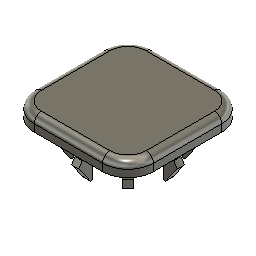
hole plug (Autodesk Fusion 360 design; units mm, degrees)
Autodesk Fusion 360 part; units mm, degrees
note: some values were not read from the file. Set by a fixed rule: which face or edge a step refers to.
sketch "Sketch1" plane through (0, 0, 0) normal (0, 1, 0) x (1, 0, 0)
  line L0 (0, 0) -> (16.4, 0)
  line L1 (16.4, 0) -> (16.4, -16.4)
  line L2 (16.4, -16.4) -> (0, -16.4)
  line L3 (0, -16.4) -> (0, 0)
  line L4 (0, 0) -> (55.9566, 0)
  line L5 (0, 0) -> (0, 56.0794)
  line L6 (-16.4, -16.4) -> (0, -16.4)
  line L7 (-16.4, 0) -> (-16.4, -16.4)
  line L8 (16.4, 0) -> (16.4, 16.4)
  line L9 (16.4, 16.4) -> (0, 16.4)
  line L10 (-16.4, 16.4) -> (0, 16.4)
  line L11 (-16.4, 0) -> (-16.4, 16.4)
  circle A0 centre (0, 0) radius 13.6
  circle A1 centre (0, 0) radius 14.6
  circle A2 centre (0, 0) radius 10.75
  line L12 (0, 0) -> (-10.3238, -10.3238) construction
  line L13 (0, 0) -> (0, -14.6) construction
  line L14 (0, 0) -> (10.3238, -10.3238) construction
  line L15 (0, 0) -> (14.6, 0) construction
  line L16 (0, 0) -> (10.3238, 10.3238) construction
  line L17 (0, 0) -> (0, 14.6) construction
  line L18 (0, 0) -> (-10.3238, 10.3238) construction
  line L19 (0, 0) -> (-14.6, 0) construction
  line L20 (-11.0066, -9.5924) -> (-8.2755, -6.8613)
  line L21 (-9.5924, -11.0066) -> (-6.8613, -8.2755)
  line L22 (1, -14.5657) -> (1, -10.7034)
  line L23 (-1, -14.5657) -> (-1, -10.7034)
  line L24 (11.0066, -9.5924) -> (8.2755, -6.8613)
  line L25 (9.5924, -11.0066) -> (6.8613, -8.2755)
  line L26 (14.5657, 1) -> (10.7034, 1)
  line L27 (14.5657, -1) -> (10.7034, -1)
  line L28 (9.5924, 11.0066) -> (6.8613, 8.2755)
  line L29 (11.0066, 9.5924) -> (8.2755, 6.8613)
  line L30 (-1, 14.5657) -> (-1, 10.7034)
  line L31 (1, 14.5657) -> (1, 10.7034)
  line L32 (-11.0066, 9.5924) -> (-8.2755, 6.8613)
  line L33 (-9.5924, 11.0066) -> (-6.8613, 8.2755)
  line L34 (-14.5657, -1) -> (-10.7034, -1)
  line L35 (-14.5657, 1) -> (-10.7034, 1)
  dimension "d3" = 32.8
  dimension "d5" = 32.8
  dimension "d6" = 27.2
  dimension "d7" = 29.2
  dimension "d8" = 21.5
  dimension "d10" = 360
  dimension "d11" = 1
  dimension "d12" = 1
  dimension "d14" = 360
  constraint horizontal L0
  constraint vertical L1
  constraint horizontal L2
  constraint vertical L3
  constraint coincident L0.start L3.end
  constraint perpendicular L3 L4
  constraint perpendicular L0 L5
  constraint symmetric L0.end L5 L7.start
  constraint symmetric L1.end L5 L6.start
  constraint symmetric L2.end L5 L3.start
  constraint symmetric L0.end L4 L1.start
  constraint symmetric L1.end L4 L8.end
  constraint symmetric L2.end L4 L9.end
  constraint symmetric L4 L6.start L10.start
  constraint symmetric L4 L2.end L9.end
  constraint symmetric L4 L7.start L11.start
  constraint concentric A0 A2
  constraint coincident A1 L12.end
  constraint coincident L3 L13.end
  constraint coincident A2 L20.end
  constraint parallel L12 L20
  constraint coincident A2 L21.end
  constraint parallel L20 L21
  constraint coincident A1 L21.start
  constraint coincident A1 L20.start
  measures "d6" diameter of A0
  measures "d7" diameter of A1
  measures "d8" diameter of A2
  measures "d11" distance of L12 L20
  measures "d12" distance of L12 L21
extrude "Extrude1" add sketch "Sketch1" along normal blind 4 makes body 1
fillet "Fillet1" radius 7 4 edges at (16.4, 2, 16.4) (-16.4, 2, 16.4) (-16.4, 2, -16.4) (16.4, 2, -16.4) on bodies 1
fillet "Fillet2" radius 2 8 edges at (14.3497, 4, -14.3497) (0, 4, -16.4) (-14.3497, 4, -14.3497) (-16.4, 4, 0) (-14.3497, 4, 14.3497) (0, 4, 16.4) (14.3497, 4, 14.3497) (16.4, 4, 0) on bodies 1
shell "Shell1" thickness 1 removed faces 1 at (5.4667, 0, 3.1333) on bodies 1
extrude "Extrude2" add sketch "Sketch1" against normal blind 12 from surface at 3 separate body contours L0 L4 A0 A2 L26 | L0 L4 A0 A2 L27 | L3 A0 A2 L22 | L3 A0 A2 L23 | L5 A0 A2 L30 | L5 A0 A2 L31 | A0 A2 L28 L29 | A0 A2 L24 L25 | A0 A2 L20 L21 | A0 A2 L32 L33 | A0 A2 L34 L35 makes body 2 at (-9.6237, -1, -8.2095) makes body 3 at (8.2095, -1, 9.6237) makes body 4 at (-1, -1, 12.6099) makes body 5 at (-1, -1, -12.6099) makes body 6 at (-12.6099, -1, 1) makes body 7 at (12.6099, -1, -1) makes body 8 at (-8.2095, -1, 9.6237) makes body 9 at (8.2095, -1, -9.6237)
extrude "Extrude4" add sketch "Sketch1" against normal blind 4 from surface at 3 contours A0 A2 L26 L29 | A0 A2 L24 L27 | A0 A2 L21 L23 | A0 A2 L22 L25 | A0 A2 L28 L31 | A0 A2 L30 L33 | A0 A2 L20 L34 | A0 A2 L32 L35 bodies 1 2 5 9 7 3 4 8 6
extrude "Extrude3" add sketch "Sketch1" along normal blind 6 from surface at -9 contours L0 L4 A0 A1 L26 | L0 L4 A0 A1 L27 | L3 A0 A1 L22 | L3 A0 A1 L23 | L5 A0 A1 L30 | L5 A0 A1 L31 | A0 A1 L28 L29 | A0 A1 L24 L25 | A0 A1 L20 L21 | A0 A1 L32 L33 | A0 A1 L34 L35 bodies 1
chamfer "Chamfer1" distance 4.5 distance2 3.25 8 edges at (-10.3238, -9, 10.3238) (14.6, -9, 0) (10.3238, -9, -10.3238) (0, -9, 14.6) (-10.3238, -9, -10.3238) (0, -9, -14.6) (10.3238, -9, 10.3238) (-14.6, -9, 0) measured on face at (-9.7589, -5, 10.8592) measured on face at (14.5996, -5, -0.1112) measured on face at (10.2448, -5, -10.4021) measured on face at (0.1112, -5, 14.5996) measured on face at (-10.8592, -5, -9.7589) measured on face at (0.5559, -5, -14.5894) measured on face at (10.4021, -5, 10.2448) measured on face at (-14.5793, -5, 0.778) on bodies 1
chamfer "Chamfer2" distance 1 distance2 1.5 8 edges at (-10.3238, -3, 10.3238) (14.6, -3, 0) (10.3238, -3, -10.3238) (0, -3, 14.6) (-10.3238, -3, -10.3238) (0, -3, -14.6) (10.3238, -3, 10.3238) (-14.6, -3, 0) measured on face at (-9.2846, -3, 10.3847) measured on face at (13.9083, -3, 0.7779) measured on face at (10.3847, -3, -9.2846) measured on face at (0.7779, -3, 13.9083) measured on face at (-9.2846, -3, -10.3847) measured on face at (0.7779, -3, -13.9083) measured on face at (10.3847, -3, 9.2846) measured on face at (-13.9083, -3, 0.7779) tangent chain off on bodies 1
combine "Combine1" [suppressed]
fillet "Fillet3" radius 1 14 edges at (1, -1, -12.1333) (7.8724, -1, -9.2866) (9.2866, -1, -7.8724) (9.2866, -1, 7.8724) (7.8724, -1, 9.2866) (1, -1, 12.1333) (-1, -1, 12.1333) (12.1333, -1, 1) (12.1333, -1, -1) (-1, -1, -12.1333) (-9.2866, -1, 7.8724) (-7.8724, -1, 9.2866) (-12.1333, -1, -1) (-12.1333, -1, 1) on bodies 1
fillet "Fillet4" radius 1 2 edges at (-12.6797, 3, 4.918) (-10.0225, 3, -3.8874) on bodies 1
extrude "Extrude5" add 1 faces at (-8.7776, -5.6308, -7.3634) along direction (-0.707107, 0, 0.707107) blind 5 and the other way blind 7 on bodies 1 bodies 1
